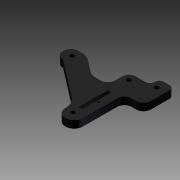
# Autodesk Inventor part: braket bawah 2
Saved by Autodesk Inventor 2012 (Build 160160000, 160)
## iProperties
Created: 2011-10-02
Part Number: braket bawah 2
Material: Default
Document SubType Name: Modeling
Designer: Yadi Irawan
Density: 1 g/cm^3
Author: Yadi Irawan
Autodesk Inventor part; units mm, degrees
ref_plane "YZ Plane" through (0, 0, 0) normal (1, 0, 0) x (0, 1, 0)
ref_plane "XZ Plane" through (0, 0, 0) normal (0, 1, 0) x (-1, 0, 0)
ref_plane "XY Plane" through (0, 0, 0) normal (0, 0, 1) x (1, 0, 0)
sketch "Sketch1" plane through (0, 0, 0) normal (0, 0, 1) x (1, 0, 0)
  line L0 (17.4112, 0) -> (20.3, 0)
  circle A0 centre (43.66, 15) radius 1.5
  circle A1 centre (-3.96, 4.8) radius 1.5
  line L1 (29.8, -3.5) -> (31.05, -3.5)
  line L2 (31.05, -23.3) -> (28.55, -23.3)
  line L3 (28.55, -23.3) -> (28.55, -3.5)
  line L4 (28.55, -3.5) -> (29.8, -3.5)
  line L5 (29.8, -23.3) -> (29.8, -28.3)
  circle A2 centre (29.8, -28.3) radius 1.5
  line L6 (31.05, -23.3) -> (31.05, -13.9)
  line L7 (31.05, -13.9) -> (33.55, -13.9)
  line L8 (33.55, -13.9) -> (33.55, -12.9)
  line L9 (33.55, -12.9) -> (31.05, -12.9)
  line L10 (31.05, -12.9) -> (31.05, -3.5)
  line L11 (36.55, -14.9) -> (36.55, -28.3)
  line L12 (49.7, 17.8) -> (49.7, 5)
  line L13 (36.55, -13) -> (36.55, -14.9)
  arc A3 (24.55, -28.3) -> (36.55, -28.3) centre (30.55, -28.3) ccw
  line L14 (24.55, -27.924) -> (24.55, -28.3)
  line L15 (5.8588, -8.6221) -> (20.6471, -19.9978)
  circle A4 centre (29.8, 9.9) radius 1.5
  arc A5 (29.8, 14.4) -> (25.3, 9.9) centre (29.8, 9.9) ccw
  line L16 (25.3, 9.9) -> (25.3, 5)
  line L17 (36.55, -13) -> (36.55, -5)
  line L18 (44.7, 0) -> (41.55, 0)
  line L19 (36.3, 14.4) -> (29.8, 14.4)
  arc A6 (36.3, 14.4) -> (39.7, 17.8) centre (36.3, 17.8) ccw
  arc A7 (41.55, 0) -> (36.55, -5) centre (41.55, -5) ccw
  arc A8 (44.7, 0) -> (49.7, 5) centre (44.7, 5) ccw
  arc A9 (20.3, 0) -> (25.3, 5) centre (20.3, 5) ccw
  arc A10 (24.55, -27.924) -> (20.6471, -19.9978) centre (14.55, -27.924) ccw
  line L20 (-3.96, 9.9) -> (-2.2612, 9.9)
  line L21 (-3.96, 9.9) -> (-5, 9.9)
  line L22 (-10, 4.9) -> (-10, 4.7)
  line L23 (11.3141, 2.0738) -> (3.8359, 7.8262)
  arc A11 (11.3141, 2.0738) -> (17.4112, 0) centre (17.4112, 10) ccw
  arc A12 (3.8359, 7.8262) -> (-2.2612, 9.9) centre (-2.2612, -0.1) ccw
  arc A13 (-5, 9.9) -> (-10, 4.9) centre (-5, 4.9) ccw
  arc A14 (-10, 4.7) -> (-5.7001, -0.2507) centre (-5, 4.7) ccw
  line L24 (5.8588, -8.6221) -> (-4.2953, -0.8401)
  arc A15 (-4.2953, -0.8401) -> (-5.7001, -0.2507) centre (-6.1202, -3.2212) ccw
  line L25 (39.7, 17.8) -> (39.7, 17.8)
  line L26 (49.7, 17.8) -> (49.7, 17.8)
  line L27 (44.7, 20.8) -> (46.7, 20.8)
  line L28 (44.7, 20.8) -> (42.7, 20.8)
  arc A16 (42.7, 20.8) -> (39.7, 17.8) centre (42.7, 17.8) ccw
  arc A17 (49.7, 17.8) -> (46.7, 20.8) centre (46.7, 17.8) ccw
  dimension "d13" = 1.25
  dimension "d15" = 2.5
  dimension "d16" = 19.8
  dimension "d17" = 5
  dimension "d25" = 9.4
  dimension "d26" = 2.5
  dimension "d27" = 1
  dimension "d70" = 5
  dimension "d71" = 5
  dimension "d72" = 10
  dimension "d79" = 10
  dimension "d80" = 5
  dimension "d83" = 3
  dimension "d85" = 3
  constraints: 58 end point, 28 point on circle, 21 tangent, 18 centre point, 4 equal radius, 2 coincident, 1 midpoint, 1 perpendicular, 1 point on line
  measures "d13" distance of L1.start L1.end
  measures "d15" distance of L2.start L2.end
  measures "d16" distance of L2.end L3.end
  measures "d17" distance of L5.start L5.end
  measures "d25" distance of L2.start L6.end
  measures "d26" distance of L6.end L7.end
  measures "d27" distance of L7.end L8.end
  measures "d70" radius of A7
  measures "d71" radius of A9
  measures "d72" radius of A10
  measures "d79" radius of A11
  measures "d80" radius of A13
  measures "d83" radius of A15
  measures "d85" radius of A16
extrude "Extrusion1" add sketch "Sketch1" along normal blind 5
body "Solid1"
